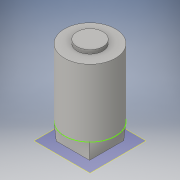
# Autodesk Inventor part: Motor
Saved by Autodesk Inventor 2016 SP2 (Build 200236200, 236)
## iProperties
Created: 2018-01-12
Part Number: Motor
Material: Generic
Document SubType Name: Modeling
Designer: CAD
Density: 1 g/cm^3
Appearance: Default
Author: CAD
Autodesk Inventor part; units mm, degrees
ref_plane "YZ Plane" through (0, 0, 0) normal (1, 0, 0) x (0, 1, 0)
ref_plane "XZ Plane" through (0, 0, 0) normal (0, 1, 0) x (-1, 0, 0)
ref_plane "XY Plane" through (0, 0, 0) normal (0, 0, 1) x (1, 0, 0)
sketch "Sketch1" plane through (0, 0, 0) normal (0, 1, 0) x (-1, 0, 0)
  circle A0 centre (0, 0) radius 16.3195
  circle A1 centre (0, 0) radius 32.131
  dimension "d0" = 32.639
  dimension "d1" = 64.262
  constraints: 2 centre point, 2 coincident
  measures "d0" diameter of A0
  measures "d1" diameter of A1
extrude "Extrusion1" add sketch "Sketch1" along normal blind 84.8868 contours A0 | A1
sketch "Sketch2" plane through (0, 84.8868, 0) normal (0, 1, 0) x (1, 0, 0)
  circle A0 centre (0, 0) radius 16.3195
  dimension "d4" = 32.639
  constraints: 1 centre point, 1 coincident
  measures "d4" diameter of A0
extrude "Extrusion2" add sketch "Sketch2" along normal blind 4.7625
sketch "Sketch3" plane through (0, 0, 0) normal (0, -1, 0) x (1, 0, 0)
  circle A0 centre (0, 0) radius 32.131
  constraints: 1 centre point, 1 coincident
ref_plane "Work Plane1" through (0, -21.463, 0) normal (0, -1, 0) x (1, 0, 0)
sketch "Sketch4" plane through (0, -21.463, 0) normal (0, -1, 0) x (1, 0, 0)
  line L0 (21.0185, 21.59) -> (-21.0185, 21.59)
  line L1 (-21.0185, 21.59) -> (-21.0185, -21.59)
  line L2 (-21.0185, -21.59) -> (21.0185, -21.59)
  line L3 (21.0185, -21.59) -> (21.0185, 21.59)
  point P0 (0, 0)
  dimension "d8" = 43.18
  dimension "d9" = 42.037
  dimension "d10" = 21.0185
  dimension "d11" = 21.59
  constraints: 8 end point, 2 parallel, 1 horizontal, 1 perpendicular
  measures "d8" distance of L2.end L0.start
  measures "d9" distance of L0.start L0.end
  measures "d10" distance from line of point (0, 0) L3
  measures "d11" distance from line of L0 point (0, 0)
loft "Loft1" add profiles "Sketch4" section 1 edges at (32.131, 0, 0)
equation "\"d10\" = 0.5 * d9"
equation "\"d11\" = 0.5 * d8"
body "Solid1"
